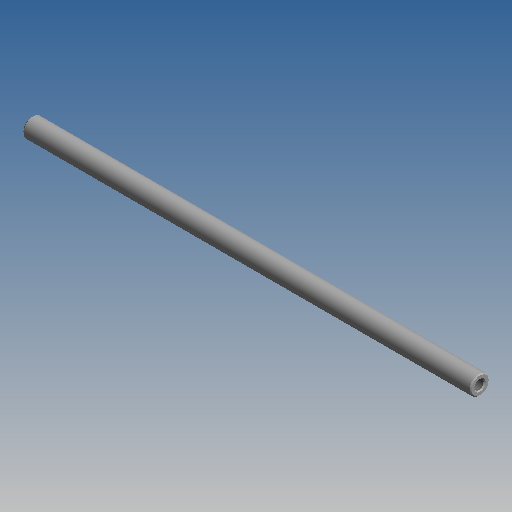
# Autodesk Inventor part: SSFMRW10-234-M6-ND6_s
Saved by Autodesk Inventor 2020 (Build 240168000, 168)
## iProperties
Part Number: SSFMRW10-234-M6-ND6_s
Material: 一般
Catalog Web Link: www.cadenas.de
Description: NSFMRW, SFMRW, PSFMRW, SSFMRW, NSFHRW, SFHRW, PSFHRW, SSFHRW, NSFRW, SFRW, PSFRW, SSFRW, HFRW, PHFRW_shaft-Rotary Shafts - Both Ends Tapped - Standard
Vendor: MISUMI
Document SubType Name: Modeling
Designer: partserver
Manufacturer: MISUMI
Mass: 17.5663 g
Surface Area: 81.2202 cm^2
Volume: 17.5663 cm^3
Density: 1 g/cm^3
Appearance: PSOLRGB-192-192-192
Category: PARTsolutions
Company: MISUMI
PSOL_IDENT_0: {$CADENAS_DATA\23d-libs\misumi\metric\11_rotary_shafts\11_components\phfrw\phfrw.prj},468 {VTYP=3D},
PSOL_IDENT_1: {NB=SSFMRW10-234-M6-ND6_s},{LINA=SSFMRW10-234-M6-ND6},{NN=NSFMRW, SFMRW, PSFMRW, SSFMRW, NSFHRW, SFH
PSOL_IDENT_2: RW, PSFHRW, SSFHRW, NSFRW, SFRW, PSFRW, SSFRW, HFRW, PHFRW_shaft},{DATE=21.06.2021 06:34:29},{GEOMDA
PSOL_IDENT_3: TE=05.02.2021 08:58:46},{VERSION=},{LINEID=30},{WBVAR=TS,MAT,ST,ALT1,L,M,N,ALT2,KC,A,WKC,C,K,E,KZ,Z,
PSOL_IDENT_4: ALT3,FC,GALT3,WFC,J,WALT3,V,ALT4,SFC,SGALT4,AG,ALT5,UC,ALT6,TA,TB,ALT31},{WBNUMERIC=L,M,N,KC,A,WKC,C
PSOL_IDENT_5: ,K,E,KZ,Z,FC,GALT3,WFC,J,WALT3,V,SFC,SGALT4,AG,UC,TA,TB}  {NB=SSFMRW10-234-M6-ND6_s},{LINA=SSFMRW10-
PSOL_IDENT_6: 234-M6-ND6},{KT=DUMMY},{PN=SSFMRW10-234-M6-ND6},{TYPE=SSFMRW},{TS=M},{TSALG= 'M','h9 (Cold-drawn)','
PSOL_IDENT_7: H','h7 (Ground)','','g6 (Ground)' },{MAT=SUS304},{MATALG= 'S45C','S45C Equivalent', 'SUS304','SUS304'
PSOL_IDENT_8: },{ST=-},{STALG= '-','-' },{D=10},{ALT1=},{L=234.0},{LALG=[15:800/0.1]},{LMINALG=15},{LMIN=15},{LMA
PSOL_IDENT_9: X=800},{M=6},{MALG=3,4,5,6},{MMIN=3},{N=6},{NALG=3,4,5,6},{NMIN=3},{NMAX=6},{NMAXD=6},{NALGMEQN=30},
PSOL_IDENT_10: {NALGMGTN=30},{NALGMLTN=30},{PITCH=1},{PITCHM=1},{ALT2=},{ALT2ALG= '', 'w/o Key Grooves','KC','with
PSOL_IDENT_11: KC (Key Groove)','WKC','with WKC (Two Key Grooves)','KCWKC','with KC + WKC (Three Key Grooves)','KZ'
PSOL_IDENT_12: ,'with KC + WKC + KZ (Four Key Grooves)' },{ALT2PN=},{KC=0.0},{KCALG=[0]},{KCMIN=0},{KCMAX=0},{A=0.0
PSOL_IDENT_13: },{AALG=[0]},{AMIN=3},{AMAX=0},{WKC=0.0},{WKCALG=[0]},{WKCMIN=0},{WKCMAX=0},{C=0.0},{CALG=[0]},{CMIN=
PSOL_IDENT_14: 3},{CMAX=0},{K=0.0},{KALG=[0]},{KMIN=0},{KMAX=229},{E=0.0},{EALG=[0]},{EMIN=3},{EMAX=100},{KZ=0.0},{
PSOL_IDENT_15: KZALG=[0]},{KZMIN=236},{KZMAX=231},{Z=0.0},{ZALG=[0]},{ZMIN=3},{ZMAX=100},{BB=0},{BBALT2=3},{TT=0.0}
PSOL_IDENT_16: ,{TTALT2=1.8},{CIFKC=1.000},{CIFWKC=1.000},{CIFK=1.000},{CIFKZ=2.000},{PCUT3D=0.000},{QCUT3D=0.000},
PSOL_IDENT_17: {ALT3=},{ALT3ALG= '', 'w/o Set Screw Flat','FC','with FC (Adds a Set Screw Flat)','WFC','with WFC (A
PSOL_IDENT_18: dds Two Set Screw Flats)','FCWFC','with FC + WFC (Adds Three Set Screw Flats)' },{ALT3PN=},{FC=0},{F
PSOL_IDENT_19: CALG=[0]},{FCMIN=0},{FCMAX=233},{GALT3=0},{GALT3ALG=[0]},{GALT3MIN=1},{GALT3MAX=70},{GALT3MAX2=70},{
PSOL_IDENT_20: GALT3MAX3=70},{WFC=0},{WFCALG=[0]},{WFCMIN=0},{WFCMIN2=2},{WFCMAX=230},{WFCMAX2=-3},{WFCMAX3=-4},{J=
PSOL_IDENT_21: 0},{JALG=[0]},{JMIN=1},{JMAX=70},{JMAX2=-2},{JMAX3=-5},{WALT3=0},{WALT3ALG=[0]},{WALT3MIN=0},{WALT3M
PSOL_IDENT_22: IN2=236},{WALT3MAX=231},{WALT3MAX2=231},{V=0},{VALG=[0]},{VMIN=1},{VMAX=70},{VMAX2=70},{CIFFC=0},{AL
PSOL_IDENT_23: T4=},{ALT4ALG= '', 'w/o SFC (2 Set Screw Flats (Angle Specified))', 'SFC'  , 'with SFC (2 Set Screw
PSOL_IDENT_24: Flats (Angle Specified))'},{ALT4PN=},{SFC=0},{SFCALG=[0]},{SFCMIN=0},{SFCMAX=233},{SGALT4=0},{SGALT4
PSOL_IDENT_25: ALG=[0]},{SGALT4MIN=1},{SGALT4MAX=70},{AG=0},{AGALG=[0]},{H=0.0},{CIFSFC=0},{ALT5=},{ALT5ALG= '', 'w
PSOL_IDENT_26: /o UC (Slit Cam Groove)', 'UC', 'with UC (Slit Cam Groove)'},{ALT5PN=},{UC=0},{UCALG=[0]},{UCMIN=1},
PSOL_IDENT_27: {UCMAX=228},{DDALT5=0},{LL1=0},{ALT6=},{ALT6ALG= '','w/o Retaining Ring Groove','TA','with TA (Retai
PSOL_IDENT_28: ning Ring Groove)','TB','with TB (Retaining Ring Groove)','TATB','with TA + TB (Two Retaining Ring G
PSOL_IDENT_29: rooves)' },{ALT6PN=},{TA=0.0},{TAALG=[0]},{TAMIN=2},{TAMAX=0},{TB=0.0},{TBALG=[0]},{TBMIN=2},{TBMAX=
PSOL_IDENT_30: 0},{DDALT6=0.0},{MM=0.00},{ALT31=ND},{ALT31ALG= '', 'w/o Tapped Depth','MD','with MD (Tapped Depth)'
PSOL_IDENT_31: ,'ND','with ND (Tapped Depth)','MDND','with MD + ND (Tapped Depth)' },{CIFALT31M=0},{CIFALT31N=0},{M
PSOL_IDENT_32: L=19},{NL=25},{ML3D1=12},{ML3D2=19},{NL3D1=18},{NL3D2=25},{CIFMN3D=0},{ERRORPN=},{ERRORMALT2=OK},{ER
PSOL_IDENT_33: RORMALT3=OK},{ERRORMALT4=OK},{ERRORMALT5=OK},{ERRORMALT6=OK},{ERRORNALT2=OK},{ERRORNALT3=OK},{ERRORN
PSOL_IDENT_34: ALT4=OK},{ERRORNALT5=OK},{ERRORNALT6=OK},{ERRORALT23=OK},{ERRORALT24=OK},{ERRORALT25=OK},{ERRORALT26=
PSOL_IDENT_35: OK},{ERRORALT34=OK},{ERRORALT35=OK},{ERRORALT36=OK},{ERRORALT45=OK},{ERRORALT46=OK},{ERRORALT56=OK}
NB: SSFMRW10-234-M6-ND6_s
NN: NSFMRW, SFMRW, PSFMRW, SSFMRW, NSFHRW, SFHRW, PSFHRW, SSFHRW, NSFRW, SFRW, PSFRW, SSFRW, HFRW, PHFRW_shaft
NT: Rotary Shafts - Both Ends Tapped - Standard
NBSYN: $PN._s
LINA: SSFMRW10-234-M6-ND6
CATALOG: Misumi
PN: SSFMRW10-234-M6-ND6
TS: h9 (Cold-drawn)
MAT: SUS304
ST: -
D: 10
ALT1: w/o LKC (Changes L Tolerance)
L: 234
M: 6
N: 6
ALT2: w/o Key Grooves
KC: 0
A: 0
WKC: 0
C: 0
K: 0
E: 0
KZ: 0
Z: 0
BB: 0
TT: 0
ALT3: w/o Set Screw Flat
FC: 0
GALT3: 0
WFC: 0
J: 0
WALT3: 0
V: 0
ALT4: w/o SFC (2 Set Screw Flats (Angle Specified))
SFC: 0
SGALT4: 0
AG: 0
H: 0
ALT5: w/o UC (Slit Cam Groove)
UC: 0
DDALT5: 0
LL1: 0
ALT6: w/o Retaining Ring Groove
TA: 0
TB: 0
DDALT6: 0
MM: 0
ALT31: with ND (Tapped Depth)
SUPPLIER: MISUMI
ARTICLENO: SSFMRW10-234-M6-ND6_s
BOMINFO: SSFMRW10-234-M6-ND6
CREATOR: CADENAS GmbH
Title: SSFMRW10-234-M6-ND6
Author: Cadenas PARTsolutions
Comments: Rotary Shafts - Both Ends Tapped - Standard
Autodesk Inventor part; units mm, degrees
ref_plane "YZ Plane" through (0, 0, 0) normal (1, 0, 0) x (0, 1, 0)
ref_plane "XZ Plane" through (0, 0, 0) normal (0, 1, 0) x (-1, 0, 0)
ref_plane "XY Plane" through (0, 0, 0) normal (0, 0, 1) x (1, 0, 0)
sketch "Sketch_1" plane through (0, 0, 0) normal (0, 0, 1) x (1, 0, 0)
  line L0 (234, 0) -> (0, 0)
  line L1 (0, 0) -> (0, 4.5)
  line L2 (0, 4.5) -> (0.5, 5)
  line L3 (0.5, 5) -> (233.5, 5)
  line L4 (233.5, 5) -> (234, 4.5)
  line L5 (234, 4.5) -> (234, 0)
  line L6 (234, 0) -> (0, 0)
  constraints: 14 end point
revolve "Revolution1" add sketch "Sketch_1" angle 360 about axis through (234, 0, 0) along (1, 0, 0)
sketch "Sketch2" plane through (0, 0, 0) normal (-1, 0, 0) x (0, 0, 1)
  point P0 (0, 0)
hole "Hole1" at (0, 0, 0) direction (1, 0, 0) diameter 4.917 depth 17.5806 tip angle 120 countersink diameter 6 countersink angle 90 thread size "M6x1" class "6H" standard "ISO Metric profile"
sketch "Sketch3" plane through (234, 0, 0) normal (1, 0, 0) x (0, 0, -1)
  point P0 (0, 0)
hole "Hole2" at (234, 0, 0) direction (-1, 0, 0) diameter 4.917 depth 23.5806 tip angle 120 countersink diameter 6 countersink angle 90 thread size "M6x1" class "6H" standard "ISO Metric profile"
body "Solid1"
